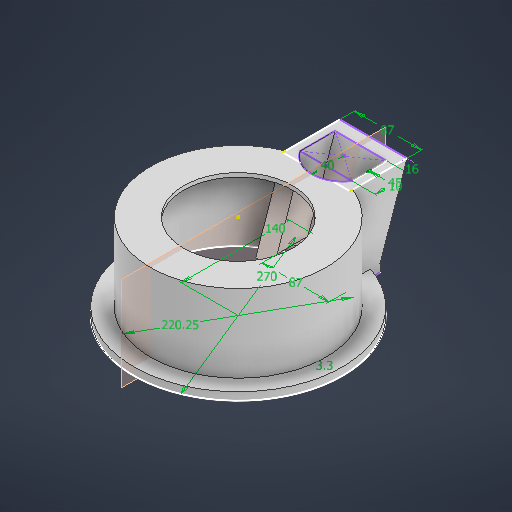
# Autodesk Inventor part: Thermal Housing
Saved by Autodesk Inventor 2026.2 (Build 302298000, 298)
## iProperties
Created: 2025-12-15
Part Number: Thermal Housing
Material: Generic
Document SubType Name: Modeling
Designer: mayhe
Density: 1 g/cm^3
Appearance: Default
Author: mayhe
Autodesk Inventor part; units mm, degrees
ref_plane "XZ Plane" through (0, 0, 0) normal (0, 1, 0) x (-1, 0, 0)
ref_plane "XY Plane" through (0, 0, 0) normal (0, 0, 1) x (1, 0, 0)
sketch "Sketch1" plane through (0, 0, 0) normal (0, 1, 0) x (-1, 0, 0)
  circle A0 centre (0, 0) radius 135
  circle A1 centre (0, 0) radius 110.125
  circle A2 centre (0, 0) radius 113.425
  line L0 (43.5, -140) -> (-43.5, -140)
  line L1 (-43.5, -140) -> (-43.5, -96.85)
  line L2 (-43.5, -96.85) -> (43.5, -96.85)
  line L3 (43.5, -96.85) -> (43.5, -140)
  point P0 (0, -135)
  point P1 (43.5, -127.7996)
  point P2 (-43.5, -127.7996)
  point P3 (43.5, -101.1695)
  point P4 (43.5, -104.752)
  point P5 (-43.5, -104.752)
  point P6 (-43.5, -101.1695)
  dimension "d0" = 270
  dimension "d1" = 220.25
  dimension "d10" = 3.3
  dimension "d17" = 87
  dimension "d38" = 140
  constraints: 8 end point, 2 centre point, 2 coincident, 2 parallel, 1 horizontal, 1 perpendicular, 3 other
  measures "d1" diameter of A1
  measures "d10" radial gap between concentric circles of A1 A2
  measures "d17" distance of L1.end L2.end
  measures "d38" distance from line of A1.centre L0
extrude "Extrusion1" add sketch "Sketch1" along normal blind 10 contours A0 L3 A2 L1 | L1 A2 L3 A0 | A0 L3 L0 L1 | L1 A1 L3 A2 | A2 L3 A1 L1
extrude "Extrusion3" add sketch "Sketch1" along normal blind 110.5 contours A2 L3 A1 L1 picked at (-78.4563, 78.6046)
sketch "Sketch4" plane through (0, 110.5, 0) normal (0, 1, 0) x (1, 0, 0)
  circle A0 centre (0, 0) radius 110.125
  circle A1 centre (0, 0) radius 70.375
  dimension "d27" = 140.75
  constraints: 2 centre point, 2 coincident
  measures "d27" diameter of A1
extrude "Extrusion7" add sketch "Sketch4" against normal blind 5
sketch "Sketch5" plane through (0, 110.5, 0) normal (0, 1, 0) x (1, 0, 0)
  line L0 (43.5, 104.752) -> (43.5, 175)
  line L1 (43.5, 175) -> (-43.5, 175)
  line L2 (-43.5, 175) -> (-43.5, 104.752)
  line L3 (-33.7867, 159) -> (33.5, 159)
  line L4 (33.5, 159) -> (33.5, 114)
  line L5 (33.5, 114) -> (-33.7867, 114)
  line L6 (-33.7867, 114) -> (-33.7867, 159)
  line L7 (-33.7867, 159) -> (33.5, 114) construction
  line L8 (33.5, 159) -> (-33.7867, 114) construction
  arc A0 (-33.7867, 114) -> (33.5, 114) centre (-0.1434, 135.6362) ccw
  line L9 (43.5, 101.1695) -> (43.5, 104.752) projected
  line L10 (43.5, 104.752) -> (43.5, 101.1695)
  line L11 (-43.5, 104.752) -> (-43.5, 101.1695) projected
  line L12 (-43.5, 101.1695) -> (-43.5, 104.752)
  line L13 (43.5, 101.1695) -> (20.1556, 101.1695)
  line L14 (-20.4423, 101.1695) -> (-43.5, 101.1695)
  point P0 (0, 0)
  point P1 (0, 113.425)
  point P2 (-0.1434, 136.5)
  dimension "d33" = 87
  dimension "d34" = 16
  dimension "d35" = 10
  dimension "d36" = 45
  dimension "d37" = 40
  constraints: 26 end point, 4 point on circle, 2 midpoint, 2 perpendicular, 1 centre point, 1 vertical
  measures "d33" distance between parallel lines of L2 L0
  measures "d34" distance between parallel lines of L1 L3
  measures "d35" distance between parallel lines of L0 L4
  measures "d36" distance of L3.end L4.end
  measures "d37" radius of A0
sketch "Sketch6" plane through (0, 0, 0) normal (1, 0, 0) x (0, 1, 0)
  line L0 (110.5, -110.125) -> (110.5, -101.1695) projected
  line L1 (110.5, -175) -> (10, -140)
  point P0 (0, 0)
  point P1 (110.5, -104.752)
  dimension "d41" = 70.248
  constraints: 2 end point
  measures "d41" distance of point (110.5, -104.752) L1.start
sweep "Sweep1" add profiles "Sketch5" path "Sketch6" keep normal constant yes path curves L1 contours L9 L13 A0 L4 L3 L6 L14 L11 L2 L1 L0
extrude "Extrusion8" cut sketch "Sketch5" against normal blind 5 contours A0 L5
body "Solid1"
